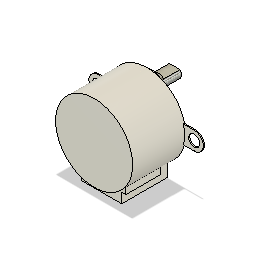
jiggler01 (Autodesk Fusion 360 archive; units mm, degrees)
design "28BYJ-48"
Autodesk Fusion 360 part; units mm, degrees
sketch "スケッチ1" plane through (0, 0, 0) normal (0, 0, 1) x (1, 0, 0)
  circle A0 centre (0, 0) radius 14
  line L0 (-40.284, 0) -> (46.998, 0) construction
  circle A1 centre (-17.5, 0) radius 2
  circle A2 centre (17.5, 0) radius 2
  circle A3 centre (17.5, 0) radius 3.3
  circle A4 centre (-17.5, 0) radius 3.3
  line L1 (-17.5, 3.3) -> (17.5, 3.3)
  line L2 (17.5, -3.3) -> (-17.5, -3.3)
  line L3 (-7.25, -11.9765) -> (7.25, -11.9765)
  line L4 (7.25, -11.9765) -> (7.25, -16.9765)
  line L5 (7.25, -16.9765) -> (-7.25, -16.9765)
  line L6 (-7.25, -16.9765) -> (-7.25, -11.9765)
  line L7 (-8.75, -10.9287) -> (8.75, -10.9287)
  line L8 (8.75, -10.9287) -> (8.75, -13.3287)
  line L9 (8.75, -13.3287) -> (-8.75, -13.3287)
  line L10 (-8.75, -13.3287) -> (-8.75, -10.9287)
  dimension "d1" = 28
  dimension "d2" = 4
  dimension "d3" = 4
  dimension "d4" = 35
  dimension "d5" = 17.5
  dimension "d6" = 1.3
  dimension "d7" = 1.3
  dimension "d8" = 14.5
  dimension "d9" = 5
  dimension "d10" = 17.5
  dimension "d11" = 2.4
  constraint coincident A0.centre origin
  constraint horizontal L0
  constraint coincident L0 A1.centre
  constraint coincident L0 A2.centre
  constraint coincident A4 L1.start
  constraint coincident A3 L1.end
  constraint coincident A3 L2.start
  constraint coincident A4 L2.end
  constraint tangent A4 L2
  constraint tangent A3 L2
  constraint tangent A3 L1
  constraint tangent A4 L1
  constraint horizontal L3
  constraint vertical L4
  constraint horizontal L5
  constraint vertical L6
  constraint coincident A0 L3.end
  constraint coincident A0 L3.start
  constraint horizontal L7
  constraint vertical L8
  constraint horizontal L9
  constraint vertical L10
  constraint coincident A0 L7.start
  constraint coincident A0 L7.end
  measures "d1" diameter of A0
  measures "d2" diameter of A1
  measures "d3" diameter of A2
  measures "d4" distance of A1.centre A2.centre
  measures "d5" distance of A0.centre A1.centre
  measures "d8" distance of L4.end L5.end
  measures "d9" distance of L3.end L4.end
  measures "d10" distance of L8.end L9.end
  measures "d11" distance of L7.start L9.end
extrude "押し出し1" add sketch "スケッチ1" along normal blind 0.4 contours A0 A4 L1 L2 | A0 A3 L1 L2 | A4 | A3 makes body 1 at (15.8685, -2.7774, 0) makes body 2 at (-15.8685, -2.7774, 0)
extrude "押し出し2" add sketch "スケッチ1" along normal blind 19.3 contours A0 L3 L7 | A0 L2 L7 | A0 L3 L9 | A0 L1 L2 | A0 L9 | A0 L1 bodies 1 2
extrude "押し出し3" add sketch "スケッチ1" along normal blind 16.5 contours A0 L6 L9 | A0 L4 L5 L6 L9 | A0 L4 L9 bodies 1
extrude "押し出し4" add sketch "スケッチ1" along normal blind 16.5 and the other way blind -4 contours A0 L6 L9 L10 | A0 L4 L8 L9 bodies 1
sketch "スケッチ2" plane through (0, 0, 0) normal (0, 0, 1) x (1, 0, 0)
  line L0 (17.5639, 8) -> (-17.5639, 8) construction
  line L1 (0, 0) -> (0, 18.0854) construction
  circle A0 centre (0, 8) radius 4.55
  circle A1 centre (0, 8) radius 2.4
  line L2 (1.9494, 9.4) -> (-1.9494, 9.4)
  line L3 (-1.9494, 6.6) -> (1.9494, 6.6)
  dimension "d22" = 8
  dimension "d23" = 9.1
  dimension "d24" = 4.8
  dimension "d25" = 2.8
  dimension "d26" = 1.4
  constraint horizontal L0
  constraint coincident L1.start origin
  constraint perpendicular L0 L1
  constraint midpoint L0 A0.centre
  constraint concentric A0 A1
  constraint coincident A1 L2.start
  constraint coincident A1 L2.end
  constraint perpendicular L1 L2
  constraint coincident A1 L3.start
  constraint coincident A1 L3.end
  constraint parallel L0 L3
  constraint coincident L1 A0.centre
  measures "d22" distance of L0 L1.start
  measures "d23" diameter of A0
  measures "d24" diameter of A1
  measures "d25" distance of L2 L3
  measures "d26" distance of L0 L2
extrude "押し出し5" add sketch "スケッチ2" against normal blind 1.7 contours A0 | A1 L2 L3 | A1 L2 | A1 L3 bodies 1
extrude "押し出し6" add sketch "スケッチ2" against normal blind 10 separate body contours A1 L2 L3 makes body 3
extrude "押し出し7" add sketch "スケッチ2" against normal blind 4 contours A1 L2 | A1 L3 bodies 3
equation "d3 = d2"
equation "d5 = d4 / 2"
equation "d26 = d25 / 2"
